Autodesk Inventor part; units mm, degrees
(part 2 of 2)
  line L890 (8.94, 31.5712) -> (9.4204, 31.2024) projected
  line L891 (8.787, 31.9019) -> (8.94, 31.5712) projected
  line L892 (8.8057, 31.9619) -> (8.787, 31.9019) projected
  line L893 (8.8181, 32.0042) -> (8.8057, 31.9619) projected
  line L894 (9.0909, 32.2844) -> (8.8181, 32.0042) projected
  line L895 (9.1333, 32.2978) -> (9.0909, 32.2844) projected
  line L896 (9.1747, 32.3122) -> (9.1333, 32.2978) projected
  line L897 (9.6789, 32.2926) -> (9.1747, 32.3122) projected
  line L898 (9.738, 32.2739) -> (9.6789, 32.2926) projected
  line L899 (9.8361, 32.244) -> (9.738, 32.2739) projected
  line L900 (10.2504, 32.0362) -> (9.8361, 32.244) projected
  line L901 (10.5617, 31.7522) -> (10.2504, 32.0362) projected
  line L902 (10.6093, 31.6838) -> (10.5617, 31.7522) projected
  line L903 (10.6556, 31.6156) -> (10.6093, 31.6838) projected
  line L904 (10.8076, 30.8229) -> (10.6556, 31.6156) projected
  line L905 (10.792, 30.733) -> (10.8076, 30.8229) projected
  line L906 (11.4372, 30.5356) -> (10.792, 30.733) projected
  line L907 (11.9632, 32.2597) -> (11.4372, 30.5356) projected
  line L908 (11.3791, 32.4385) -> (11.9632, 32.2597) projected
  line L909 (11.1374, 32.148) -> (11.3791, 32.4385) projected
  line L910 (11.1042, 32.1945) -> (11.1374, 32.148) projected
  line L911 (10.6712, 32.5965) -> (11.1042, 32.1945) projected
  line L912 (10.6185, 32.6306) -> (10.6712, 32.5965) projected
  line L913 (10.5647, 32.6647) -> (10.6185, 32.6306) projected
  line L914 (9.9148, 32.9531) -> (10.5647, 32.6647) projected
  line L915 (9.8393, 32.9757) -> (9.9148, 32.9531) projected
  line L916 (9.6862, 33.0224) -> (9.8393, 32.9757) projected
  line L917 (8.9948, 33.1245) -> (9.6862, 33.0224) projected
  line L918 (8.4016, 33.0533) -> (8.9948, 33.1245) projected
  line L919 (8.2982, 33.0129) -> (8.4016, 33.0533) projected
  line L920 (8.1938, 32.9736) -> (8.2982, 33.0129) projected
  line L921 (7.7764, 32.6544) -> (8.1938, 32.9736) projected
  line L922 (7.4929, 32.1768) -> (7.7764, 32.6544) projected
  line L923 (7.4569, 32.057) -> (7.4929, 32.1768) projected
  line L924 (7.4404, 32.0053) -> (7.4569, 32.057) projected
  line L925 (7.3981, 31.4999) -> (7.4404, 32.0053) projected
  line L926 (7.4051, 31.4502) -> (7.3981, 31.4999) projected
  line L927 (7.4125, 31.4018) -> (7.4051, 31.4502) projected
  line L928 (7.5985, 30.9406) -> (7.4125, 31.4018) projected
  line L929 (7.6295, 30.8972) -> (7.5985, 30.9406) projected
  line L930 (7.6522, 30.8642) -> (7.6295, 30.8972) projected
  line L931 (7.9766, 30.5284) -> (7.6522, 30.8642) projected
  line L932 (8.0181, 30.4943) -> (7.9766, 30.5284) projected
  line L933 (8.0595, 30.4611) -> (8.0181, 30.4943) projected
  line L934 (8.3746, 30.2442) -> (8.0595, 30.4611) projected
  line L935 (8.8365, 29.9609) -> (8.3746, 30.2442) projected
  line L936 (8.9514, 29.8936) -> (8.8365, 29.9609) projected
  line L937 (8.9628, 29.8875) -> (8.9514, 29.8936) projected
  line L938 (9.1249, 29.7934) -> (8.9628, 29.8875) projected
  line L939 (9.1467, 29.7812) -> (9.1249, 29.7934) projected
  line L940 (9.2772, 29.7056) -> (9.1467, 29.7812) projected
  line L941 (9.7039, 29.3399) -> (9.2772, 29.7056) projected
  line L942 (9.8279, 28.9874) -> (9.7039, 29.3399) projected
  line L943 (9.8071, 28.9192) -> (9.8279, 28.9874) projected
  line L944 (9.7938, 28.8758) -> (9.8071, 28.9192) projected
  line L945 (9.5, 28.5906) -> (9.7938, 28.8758) projected
  line L946 (9.4094, 28.5636) -> (9.5, 28.5906) projected
  line L947 (8.8489, 28.5967) -> (9.4094, 28.5636) projected
  line L948 (8.7828, 28.6163) -> (8.8489, 28.5967) projected
  line L949 (8.6857, 28.6464) -> (8.7828, 28.6163) projected
  line L950 (8.2736, 28.8644) -> (8.6857, 28.6464) projected
  line L951 (7.956, 29.1764) -> (8.2736, 28.8644) projected
  line L952 (7.9077, 29.2532) -> (7.956, 29.1764) projected
  line L953 (7.8579, 29.3303) -> (7.9077, 29.2532) projected
  line L954 (7.6853, 30.208) -> (7.8579, 29.3303) projected
  line L955 (7.6998, 30.3063) -> (7.6853, 30.208) projected
  line L956 (7.0683, 30.4985) -> (7.6998, 30.3063) projected
  line L957 (6.502, 28.6443) -> (7.0683, 30.4985) projected
  line L958 (-1.8759, 29.4062) -> (-1.8602, 30.0519) projected
  line L959 (2.9983, 29.2869) -> (-1.8759, 29.4062) projected
  line L960 (3.048, 31.3222) -> (2.9983, 29.2869) projected
  line L961 (2.4018, 31.3374) -> (3.048, 31.3222) projected
  line L962 (2.3845, 31.2003) -> (2.4018, 31.3374) projected
  line L963 (2.2521, 30.6494) -> (2.3845, 31.2003) projected
  line L964 (2.0559, 30.2834) -> (2.2521, 30.6494) projected
  line L965 (2.0071, 30.2379) -> (2.0559, 30.2834) projected
  line L966 (1.9585, 30.1923) -> (2.0071, 30.2379) projected
  line L967 (1.5853, 30.0384) -> (1.9585, 30.1923) projected
  line L968 (1.0388, 29.9815) -> (1.5853, 30.0384) projected
  line L969 (0.9034, 29.9847) -> (1.0388, 29.9815) projected
  line L970 (0.2429, 30.0013) -> (0.9034, 29.9847) projected
  line L971 (0.2821, 31.5908) -> (0.2429, 30.0013) projected
  line L972 (0.4041, 31.5878) -> (0.2821, 31.5908) projected
  line L973 (0.4743, 31.5868) -> (0.4041, 31.5878) projected
  line L974 (0.9293, 31.447) -> (0.4743, 31.5868) projected
  line L975 (0.9498, 31.4203) -> (0.9293, 31.447) projected
  line L976 (0.9695, 31.3944) -> (0.9498, 31.4203) projected
  line L977 (1.0697, 30.8343) -> (0.9695, 31.3944) projected
  line L978 (1.0697, 30.7486) -> (1.0697, 30.8343) projected
  line L979 (1.6867, 30.7299) -> (1.0697, 30.7486) projected
  line L980 (1.7425, 32.9809) -> (1.6867, 30.7299) projected
  line L981 (1.1245, 32.9954) -> (1.7425, 32.9809) projected
  line L982 (1.1224, 32.9178) -> (1.1245, 32.9954) projected
  line L983 (0.9942, 32.4012) -> (1.1224, 32.9178) projected
  line L984 (0.9715, 32.3753) -> (0.9942, 32.4012) projected
  line L985 (0.9477, 32.3505) -> (0.9715, 32.3753) projected
  line L986 (0.4879, 32.2326) -> (0.9477, 32.3505) projected
  line L987 (0.4206, 32.2337) -> (0.4879, 32.2326) projected
  line L988 (0.2987, 32.2368) -> (0.4206, 32.2337) projected
  line L989 (0.3328, 33.6404) -> (0.2987, 32.2368) projected
  line L990 (0.9715, 33.6248) -> (0.3328, 33.6404) projected
  line L991 (1.0636, 33.6227) -> (0.9715, 33.6248) projected
  line L992 (1.7052, 33.5619) -> (1.0636, 33.6227) projected
  line L993 (1.7416, 33.5516) -> (1.7052, 33.5619) projected
  line L994 (1.7766, 33.5421) -> (1.7416, 33.5516) projected
  line L995 (2.0662, 33.383) -> (1.7766, 33.5421) projected
  line L996 (2.0888, 33.3602) -> (2.0662, 33.383) projected
  line L997 (2.1105, 33.3396) -> (2.0888, 33.3602) projected
  line L998 (2.2862, 33.0451) -> (2.1105, 33.3396) projected
  line L999 (2.2995, 33.0077) -> (2.2862, 33.0451) projected
  line L1000 (2.3119, 32.9715) -> (2.2995, 33.0077) projected
  line L1001 (2.4186, 32.426) -> (2.3119, 32.9715) projected
  line L1002 (2.4268, 32.3536) -> (2.4186, 32.426) projected
  line L1003 (3.0737, 32.3372) -> (2.4268, 32.3536) projected
  line L1004 (3.1192, 34.218) -> (3.0737, 32.3372) projected
  line L1005 (-1.7549, 34.3378) -> (3.1192, 34.218) projected
  line L1006 (-1.7703, 33.692) -> (-1.7549, 34.3378) projected
  line L1007 (-1.4987, 33.685) -> (-1.7703, 33.692) projected
  line L1008 (-1.451, 33.6838) -> (-1.4987, 33.685) projected
  line L1009 (-1.1451, 33.6187) -> (-1.451, 33.6838) projected
  line L1010 (-1.1316, 33.6063) -> (-1.1451, 33.6187) projected
  line L1011 (-1.1192, 33.5949) -> (-1.1316, 33.6063) projected
  line L1012 (-1.0594, 33.2952) -> (-1.1192, 33.5949) projected
  line L1013 (-1.0605, 33.2464) -> (-1.0594, 33.2952) projected
  line L1014 (-1.1287, 30.4611) -> (-1.0605, 33.2464) projected
  line L1015 (-1.1299, 30.4147) -> (-1.1287, 30.4611) projected
  line L1016 (-1.2042, 30.1201) -> (-1.1299, 30.4147) projected
  line L1017 (-1.2177, 30.1078) -> (-1.2042, 30.1201) projected
  line L1018 (-1.232, 30.0963) -> (-1.2177, 30.1078) projected
  line L1019 (-1.5398, 30.0447) -> (-1.232, 30.0963) projected
  line L1020 (-1.5874, 30.0459) -> (-1.5398, 30.0447) projected
  line L1021 (-1.8602, 30.0519) -> (-1.5874, 30.0459) projected
  line L1022 (-10.0222, 28.8167) -> (-10.7488, 31.5072) projected
  line L1023 (-10.0108, 28.7724) -> (-10.0222, 28.8167) projected
  line L1024 (-10.0005, 28.4697) -> (-10.0108, 28.7724) projected
  line L1025 (-10.0096, 28.454) -> (-10.0005, 28.4697) projected
  line L1026 (-10.0201, 28.4396) -> (-10.0096, 28.454) projected
  line L1027 (-10.3053, 28.3001) -> (-10.0201, 28.4396) projected
  line L1028 (-10.3518, 28.2866) -> (-10.3053, 28.3001) projected
  line L1029 (-10.6008, 28.2184) -> (-10.3518, 28.2866) projected
  line L1030 (-10.4325, 27.5953) -> (-10.6008, 28.2184) projected
  line L1031 (-8.2309, 28.1885) -> (-10.4325, 27.5953) projected
  line L1032 (-8.3995, 28.8126) -> (-8.2309, 28.1885) projected
  line L1033 (-8.6704, 28.7394) -> (-8.3995, 28.8126) projected
  line L1034 (-8.7177, 28.7268) -> (-8.6704, 28.7394) projected
  line L1035 (-9.0343, 28.7051) -> (-8.7177, 28.7268) projected
  line L1036 (-9.0495, 28.7133) -> (-9.0343, 28.7051) projected
  line L1037 (-9.0663, 28.7219) -> (-9.0495, 28.7133) projected
  line L1038 (-9.2099, 28.9886) -> (-9.0663, 28.7219) projected
  line L1039 (-9.2213, 29.0328) -> (-9.2099, 28.9886) projected
  line L1040 (-9.897, 31.5401) -> (-9.2213, 29.0328) projected
  line L1041 (-6.9908, 28.5234) -> (-9.897, 31.5401) projected
  line L1042 (-5.5274, 28.9181) -> (-6.9908, 28.5234) projected
  line L1043 (-6.5328, 32.6441) -> (-5.5274, 28.9181) projected
  line L1044 (-6.5452, 32.6896) -> (-6.5328, 32.6441) projected
  line L1045 (-6.5555, 32.9923) -> (-6.5452, 32.6896) projected
  line L1046 (-6.5452, 33.0077) -> (-6.5555, 32.9923) projected
  line L1047 (-6.5361, 33.0234) -> (-6.5452, 33.0077) projected
  line L1048 (-6.2507, 33.1628) -> (-6.5361, 33.0234) projected
  line L1049 (-6.2031, 33.1754) -> (-6.2507, 33.1628) projected
  line L1050 (-5.9819, 33.2352) -> (-6.2031, 33.1754) projected
  line L1051 (-6.1505, 33.8595) -> (-5.9819, 33.2352) projected
  line L1052 (-8.3241, 33.2735) -> (-6.1505, 33.8595) projected
  line L1053 (-8.1555, 32.649) -> (-8.3241, 33.2735) projected
  line L1054 (-7.8848, 32.7216) -> (-8.1555, 32.649) projected
  line L1055 (-7.8383, 32.7349) -> (-7.8848, 32.7216) projected
  line L1056 (-7.5221, 32.7567) -> (-7.8383, 32.7349) projected
  line L1057 (-7.5055, 32.7483) -> (-7.5221, 32.7567) projected
  line L1058 (-7.4889, 32.7401) -> (-7.5055, 32.7483) projected
  line L1059 (-7.3464, 32.4734) -> (-7.4889, 32.7401) projected
  line L1060 (-7.3341, 32.4281) -> (-7.3464, 32.4734) projected
  line L1061 (-6.718, 30.144) -> (-7.3341, 32.4281) projected
  line L1062 (-9.4404, 32.9715) -> (-6.718, 30.144) projected
  line L1063 (-11.7171, 32.3578) -> (-9.4404, 32.9715) projected
  line L1064 (-11.5496, 31.7337) -> (-11.7171, 32.3578) projected
  line L1065 (-11.2995, 31.8005) -> (-11.5496, 31.7337) projected
  line L1066 (-11.253, 31.8141) -> (-11.2995, 31.8005) projected
  line L1067 (-10.9368, 31.8358) -> (-11.253, 31.8141) projected
  line L1068 (-10.9202, 31.8265) -> (-10.9368, 31.8358) projected
  line L1069 (-10.9036, 31.8194) -> (-10.9202, 31.8265) projected
  line L1070 (-10.7612, 31.5527) -> (-10.9036, 31.8194) projected
  line L1071 (-10.7488, 31.5072) -> (-10.7612, 31.5527) projected
  line L1072 (-19.5141, 26.9626) -> (-19.5389, 27.0032) projected
  line L1073 (-18.0278, 24.6063) -> (-19.5141, 26.9626) projected
  line L1074 (-18.003, 24.5671) -> (-18.0278, 24.6063) projected
  line L1075 (-17.9049, 24.2807) -> (-18.003, 24.5671) projected
  line L1076 (-17.9089, 24.263) -> (-17.9049, 24.2807) projected
  line L1077 (-17.9142, 24.2457) -> (-17.9089, 24.263) projected
  line L1078 (-18.1457, 24.0276) -> (-17.9142, 24.2457) projected
  line L1079 (-18.1859, 24.0017) -> (-18.1457, 24.0276) projected
  line L1080 (-18.4052, 23.8641) -> (-18.1859, 24.0017) projected
  line L1081 (-18.0598, 23.3174) -> (-18.4052, 23.8641) projected
  line L1082 (-16.1313, 24.533) -> (-18.0598, 23.3174) projected
  line L1083 (-16.4765, 25.0795) -> (-16.1313, 24.533) projected
  line L1084 (-16.7131, 24.9298) -> (-16.4765, 25.0795) projected
  line L1085 (-16.7545, 24.905) -> (-16.7131, 24.9298) projected
  line L1086 (-17.0511, 24.7901) -> (-16.7545, 24.905) projected
  line L1087 (-17.0688, 24.7934) -> (-17.0511, 24.7901) projected
  line L1088 (-17.0873, 24.7964) -> (-17.0688, 24.7934) projected
  line L1089 (-17.3012, 25.0092) -> (-17.0873, 24.7964) projected
  line L1090 (-17.3262, 25.0487) -> (-17.3012, 25.0092) projected
  line L1091 (-18.7109, 27.2438) -> (-17.3262, 25.0487) projected
  line L1092 (-15.044, 25.219) -> (-18.7109, 27.2438) projected
  line L1093 (-13.7625, 26.0263) -> (-15.044, 25.219) projected
  line L1094 (-15.8212, 29.2913) -> (-13.7625, 26.0263) projected
  line L1095 (-15.846, 29.3315) -> (-15.8212, 29.2913) projected
  line L1096 (-15.9452, 29.6168) -> (-15.846, 29.3315) projected
  line L1097 (-15.9401, 29.6344) -> (-15.9452, 29.6168) projected
  line L1098 (-15.9349, 29.6528) -> (-15.9401, 29.6344) projected
  line L1099 (-15.7044, 29.8702) -> (-15.9349, 29.6528) projected
  line L1100 (-15.6631, 29.8957) -> (-15.7044, 29.8702) projected
  line L1101 (-15.4688, 30.0188) -> (-15.6631, 29.8957) projected
  line L1102 (-15.813, 30.5655) -> (-15.4688, 30.0188) projected
  line L1103 (-17.7178, 29.3644) -> (-15.813, 30.5655) projected
  line L1104 (-17.3736, 28.8179) -> (-17.7178, 29.3644) projected
  line L1105 (-17.137, 28.9676) -> (-17.3736, 28.8179) projected
  line L1106 (-17.0966, 28.9935) -> (-17.137, 28.9676) projected
  line L1107 (-16.8, 29.1073) -> (-17.0966, 28.9935) projected
  line L1108 (-16.7813, 29.1042) -> (-16.8, 29.1073) projected
  line L1109 (-16.7638, 29.101) -> (-16.7813, 29.1042) projected
  line L1110 (-16.5478, 28.8893) -> (-16.7638, 29.101) projected
  line L1111 (-16.523, 28.8489) -> (-16.5478, 28.8893) projected
  line L1112 (-15.2611, 26.847) -> (-16.523, 28.8489) projected
  line L1113 (-18.6955, 28.7476) -> (-15.2611, 26.847) projected
  line L1114 (-20.6912, 27.4897) -> (-18.6955, 28.7476) projected
  line L1115 (-20.346, 26.943) -> (-20.6912, 27.4897) projected
  line L1116 (-20.128, 27.0815) -> (-20.346, 26.943) projected
  line L1117 (-20.0877, 27.1074) -> (-20.128, 27.0815) projected
  line L1118 (-19.791, 27.2211) -> (-20.0877, 27.1074) projected
  line L1119 (-19.7725, 27.2179) -> (-19.791, 27.2211) projected
  line L1120 (-19.7549, 27.2148) -> (-19.7725, 27.2179) projected
  line L1121 (-19.5389, 27.0032) -> (-19.7549, 27.2148) projected
  line L1122 (-29.9114, 16.9404) -> (-28.1947, 16.1199) projected
  line L1123 (-31.9825, 12.61) -> (-29.9114, 16.9404) projected
  line L1124 (-30.2658, 11.7885) -> (-31.9825, 12.61) projected
  line L1125 (-29.9806, 12.3859) -> (-30.2658, 11.7885) projected
  line L1126 (-30.0757, 12.4313) -> (-29.9806, 12.3859) projected
  line L1127 (-30.6937, 12.95) -> (-30.0757, 12.4313) projected
  line L1128 (-30.7216, 13.0079) -> (-30.6937, 12.95) projected
  line L1129 (-30.7506, 13.067) -> (-30.7216, 13.0079) projected
  line L1130 (-30.7123, 13.7366) -> (-30.7506, 13.067) projected
  line L1131 (-30.6762, 13.812) -> (-30.7123, 13.7366) projected
  line L1132 (-30.6451, 13.8772) -> (-30.6762, 13.812) projected
  line L1133 (-27.898, 12.5635) -> (-30.6451, 13.8772) projected
  line L1134 (-27.8102, 12.5212) -> (-27.898, 12.5635) projected
  line L1135 (-27.773, 12.5037) -> (-27.8102, 12.5212) projected
  line L1136 (-27.5353, 12.3671) -> (-27.773, 12.5037) projected
  line L1137 (-27.5249, 12.3568) -> (-27.5353, 12.3671) projected
  line L1138 (-27.5146, 12.3476) -> (-27.5249, 12.3568) projected
  line L1139 (-27.4702, 12.2431) -> (-27.5146, 12.3476) projected
  line L1140 (-27.4712, 12.2316) -> (-27.4702, 12.2431) projected
  line L1141 (-27.4743, 12.2131) -> (-27.4712, 12.2316) projected
  line L1142 (-27.5332, 11.988) -> (-27.4743, 12.2131) projected
  line L1143 (-27.5425, 11.9611) -> (-27.5332, 11.988) projected
  line L1144 (-27.5528, 11.935) -> (-27.5425, 11.9611) projected
  line L1145 (-27.6831, 11.6323) -> (-27.5528, 11.935) projected
  line L1146 (-27.6996, 11.5973) -> (-27.6831, 11.6323) projected
  line L1147 (-27.1291, 11.3245) -> (-27.6996, 11.5973) projected
  line L1148 (-25.8672, 13.9638) -> (-27.1291, 11.3245) projected
  line L1149 (-26.4377, 14.237) -> (-25.8672, 13.9638) projected
  line L1150 (-26.4625, 14.1882) -> (-26.4377, 14.237) projected
  line L1151 (-26.6423, 13.8534) -> (-26.4625, 14.1882) projected
  line L1152 (-26.6537, 13.8349) -> (-26.6423, 13.8534) projected
  line L1153 (-26.665, 13.8173) -> (-26.6537, 13.8349) projected
  line L1154 (-26.7736, 13.6787) -> (-26.665, 13.8173) projected
  line L1155 (-26.7839, 13.6695) -> (-26.7736, 13.6787) projected
  line L1156 (-26.7921, 13.6611) -> (-26.7839, 13.6695) projected
  line L1157 (-26.9028, 13.6282) -> (-26.7921, 13.6611) projected
  line L1158 (-26.9162, 13.6291) -> (-26.9028, 13.6282) projected
  line L1159 (-26.9307, 13.6322) -> (-26.9162, 13.6291) projected
  line L1160 (-27.1911, 13.7345) -> (-26.9307, 13.6322) projected
  line L1161 (-27.2294, 13.7522) -> (-27.1911, 13.7345) projected
  line L1162 (-30.0571, 15.104) -> (-27.2294, 13.7522) projected
  line L1163 (-30.025, 15.1722) -> (-30.0571, 15.104) projected
  line L1164 (-29.9899, 15.2476) -> (-30.025, 15.1722) projected
  line L1165 (-29.7698, 15.5307) -> (-29.9899, 15.2476) projected
  line L1166 (-29.4969, 15.6932) -> (-29.7698, 15.5307) projected
  line L1167 (-29.4339, 15.7065) -> (-29.4969, 15.6932) projected
  line L1168 (-29.3708, 15.721) -> (-29.4339, 15.7065) projected
  line L1169 (-29.008, 15.7025) -> (-29.3708, 15.721) projected
  line L1170 (-28.5791, 15.5638) -> (-29.008, 15.7025) projected
  line L1171 (-28.483, 15.5174) -> (-28.5791, 15.5638) projected
  line L1172 (-28.1947, 16.1199) -> (-28.483, 15.5174) projected
  line L1173 (-23.8011, 17.3778) -> (-24.2869, 17.8047) projected
  line L1174 (-20.5869, 21.0436) -> (-23.8011, 17.3778) projected
  line L1175 (-22.1175, 22.386) -> (-20.5869, 21.0436) projected
  line L1176 (-22.5433, 21.9003) -> (-22.1175, 22.386) projected
  line L1177 (-22.4493, 21.7993) -> (-22.5433, 21.9003) projected
  line L1178 (-22.1113, 21.3444) -> (-22.4493, 21.7993) projected
  line L1179 (-21.9563, 20.959) -> (-22.1113, 21.3444) projected
  line L1180 (-21.9521, 20.8918) -> (-21.9563, 20.959) projected
  line L1181 (-21.949, 20.8257) -> (-21.9521, 20.8918) projected
  line L1182 (-22.0689, 20.4412) -> (-21.949, 20.8257) projected
  line L1183 (-22.3759, 19.9854) -> (-22.0689, 20.4412) projected
  line L1184 (-22.4648, 19.8829) -> (-22.3759, 19.9854) projected
  line L1185 (-22.8999, 19.386) -> (-22.4648, 19.8829) projected
  line L1186 (-24.0957, 20.4338) -> (-22.8999, 19.386) projected
  line L1187 (-24.0161, 20.5258) -> (-24.0957, 20.4338) projected
  line L1188 (-23.9696, 20.5795) -> (-24.0161, 20.5258) projected
  line L1189 (-23.5706, 20.8392) -> (-23.9696, 20.5795) projected
  line L1190 (-23.5376, 20.838) -> (-23.5706, 20.8392) projected
  line L1191 (-23.5045, 20.8371) -> (-23.5376, 20.838) projected
  line L1192 (-23.0115, 20.5557) -> (-23.5045, 20.8371) projected
  line L1193 (-22.9454, 20.4999) -> (-23.0115, 20.5557) projected
  line L1194 (-22.5351, 20.9622) -> (-22.9454, 20.4999) projected
  line L1195 (-24.228, 22.4462) -> (-22.5351, 20.9622) projected
  line L1196 (-24.6352, 21.981) -> (-24.228, 22.4462) projected
  line L1197 (-24.5763, 21.9306) -> (-24.6352, 21.981) projected
  line L1198 (-24.2611, 21.5006) -> (-24.5763, 21.9306) projected
  line L1199 (-24.2559, 21.4653) -> (-24.2611, 21.5006) projected
  line L1200 (-24.2518, 21.4312) -> (-24.2559, 21.4653) projected
  line L1201 (-24.4564, 21.0045) -> (-24.2518, 21.4312) projected
  line L1202 (-24.5008, 20.9525) -> (-24.4564, 21.0045) projected
  line L1203 (-24.5814, 20.8609) -> (-24.5008, 20.9525) projected
  line L1204 (-25.6367, 21.7869) -> (-24.5814, 20.8609) projected
  line L1205 (-25.216, 22.2662) -> (-25.6367, 21.7869) projected
  line L1206 (-25.155, 22.3367) -> (-25.216, 22.2662) projected
  line L1207 (-24.6972, 22.7905) -> (-25.155, 22.3367) projected
  line L1208 (-24.6662, 22.811) -> (-24.6972, 22.7905) projected
  line L1209 (-24.6362, 22.8328) -> (-24.6662, 22.811) projected
  line L1210 (-24.3282, 22.9537) -> (-24.6362, 22.8328) projected
  line L1211 (-24.2972, 22.9558) -> (-24.3282, 22.9537) projected
  line L1212 (-24.2672, 22.9587) -> (-24.2972, 22.9558) projected
  line L1213 (-23.9293, 22.9061) -> (-24.2672, 22.9587) projected
  line L1214 (-23.8921, 22.8918) -> (-23.9293, 22.9061) projected
  line L1215 (-23.8559, 22.8783) -> (-23.8921, 22.8918) projected
  line L1216 (-23.3681, 22.6104) -> (-23.8559, 22.8783) projected
  line L1217 (-23.3071, 22.5702) -> (-23.3681, 22.6104) projected
  line L1218 (-22.8813, 23.056) -> (-23.3071, 22.5702) projected
  line L1219 (-24.2962, 24.2962) -> (-22.8813, 23.056) projected
  line L1220 (-27.5105, 20.6304) -> (-24.2962, 24.2962) projected
  line L1221 (-27.0237, 20.2044) -> (-27.5105, 20.6304) projected
  line L1222 (-26.8449, 20.4092) -> (-27.0237, 20.2044) projected
  line L1223 (-26.8138, 20.4452) -> (-26.8449, 20.4092) projected
  line L1224 (-26.5669, 20.6374) -> (-26.8138, 20.4452) projected
  line L1225 (-26.5493, 20.6395) -> (-26.5669, 20.6374) projected
  line L1226 (-26.5317, 20.6428) -> (-26.5493, 20.6395) projected
  line L1227 (-26.263, 20.497) -> (-26.5317, 20.6428) projected
  line L1228 (-26.2268, 20.465) -> (-26.263, 20.497) projected
  line L1229 (-24.1329, 18.6282) -> (-26.2268, 20.465) projected
  line L1230 (-24.0978, 18.5974) -> (-24.1329, 18.6282) projected
  line L1231 (-23.919, 18.3512) -> (-24.0978, 18.5974) projected
  line L1232 (-23.9179, 18.3328) -> (-23.919, 18.3512) projected
  line L1233 (-24.0761, 18.0453) -> (-23.9179, 18.3328) projected
  line L1234 (-24.1071, 18.0091) -> (-24.0761, 18.0453) projected
  line L1235 (-24.2869, 17.8047) -> (-24.1071, 18.0091) projected
  point P0 (0, 0)
body "Solid1"
